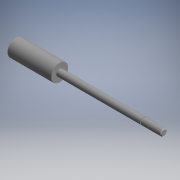
# Autodesk Inventor part: 0070.725-R0000_rod
Saved by Autodesk Inventor 2017.3 (Build 213256000, 256)
## iProperties
Part Number: 0070.725-R0000_rod
Material: Generic
Catalog Web Link: www.cadenas.de
Description: Standard Air Cylinder_rod-Original Line - Standard Air Cylinders
Vendor: BIMBA
Document SubType Name: Modeling
Designer: partserver
Manufacturer: BIMBA
Mass: 1.45088 g
Surface Area: 11.2381 cm^2
Volume: 1.45088 cm^3
Density: 1 g/cm^3
Appearance: PSOLRGB-181-181-181
Category: PARTsolutions
Company: BIMBA
Title: 0070.725-R0000_rod
Author: Cadenas PARTsolutions
Comments: Original Line - Standard Air Cylinders
PSOL_IDENT_0: {$CADENAS_DATA\23d-libs\bimba\bimba_brand\bimba_imperial\bimba_full_line\original_line_cylinders\sta
PSOL_IDENT_1: ndard_air_cylinders\rod.prj},337 {VTYP=3D},{NB=0070.725-R0000_rod},{LINA=0070.725-R0000_rod},{NN=Sta
PSOL_IDENT_2: ndard Air Cylinder_rod},{DATE=19.01.2022 10:19:37},{GEOMDATE=27.08.2019 11:00:52},{VERSION=},{LINEID=
PSOL_IDENT_3: 20},{WBVAR=STROKE,ACTING,MNT,DER,NR,BM,CO,M,EE,EEL,K,Q,Y,F,G,T,B,H,SER,SR,NT,W,E,HL,ST,STP,PRC,PB,CO
PSOL_IDENT_4: LOR1,FCD,RCD,BCD,ZHJ},{WBNUMERIC=STROKE,EEL,COLOR1,FCD,RCD,BCD,ZHJ}  {NB=0070.725-R0000_rod},{LINA=0
PSOL_IDENT_5: 070.725-R0000_rod},{KT=DUMMY},{PN=0070.725-R000},{DASH=-},{BORE=0.31250000},{BOREPN=007},{STROKE=0.7
PSOL_IDENT_6: 25},{STROKEALG=[0.001:50/0.001]},{STROKE1=0.725},{ACTING=R},{ACTINGALG= '' , 'Single Acting' , 'R' ,
PSOL_IDENT_7: 'Reverse Single Acting' , 'D' , 'Double Acting' },{ACTINGPN=R},{MNT=},{MNTALG= '' , 'Front Nose Mou
PSOL_IDENT_8: nting' , 'P' , 'Rear Pivot Mounting' },{TYPE=},{MNTPN=},{DER=},{DERALG= '' , 'N/A' },{NR=},{NRALG= ''
PSOL_IDENT_9: , 'N/A' },{NRPN=},{BM=},{BMALG= '' , 'N/A' },{BMPN=},{CO=},{COALG= '' , 'N/A' },{M=},{MALG= '', 'Wi
PSOL_IDENT_10: thout Magnet', 'M', 'With Magnet' },{EE=},{EEL=0},{EEMAX=49},{EEALG= '', 'Without Extra Extension', '
PSOL_IDENT_11: EE', 'With Extra Extension' },{EELALG=0},{EEPN=},{EEPN1=0.000},{K=},{KALG= '' , 'N/A' },{KPN=},{Q=},
PSOL_IDENT_12: {QALG= '' , 'Without Side Ported Rear Head' , 'Q' , 'With Side Ported Rear Head' },{QPN=},{Y=},{YALG=
PSOL_IDENT_13: '' , 'N/A' },{YPN=},{F=},{FALG= '', 'Standard', 'F', 'Molycoated Body' },{FPN=},{G=},{GPN=},{T=},{T
PSOL_IDENT_14: ALG= '' , 'Standard' , 'N' , 'Low Temperature' , 'V' , 'High Temperature' },{NPN=},{VPN=},{B=},{BALG=
PSOL_IDENT_15: '' , 'With Bumper' },{BPN=},{H=},{HALG= '', 'N/A' },{HPN=},{SER=},{SERALG= '' , 'N/A' },{SR=},{SRAL
PSOL_IDENT_16: G= 'C' , 'Carbon Steel Rod' , 'SR' , '303 Stainless Steel Rod' , '' , '303 Stainless Steel Rod1' },{
PSOL_IDENT_17: SRPN=},{SRCON=0},{NT=},{NTPN=},{W=},{WALG= '' , 'Without Wiper' , 'W' , 'With Wiper' },{WPN=},{E=},{
PSOL_IDENT_18: EALG= '' , 'Without Special Lube and Seals' , 'E' , 'With Special Lube and Seals' },{EPN=},{HL=},{HL
PSOL_IDENT_19: ALG= '' , 'N/A' },{ST=},{STALG= '' , 'Without Switch Track' , 'T' , 'With Switch Track' },{STP=},{ST
PSOL_IDENT_20: PALG= '' , 'N/A' },{STPN=},{PRC=},{PRCALG= '' , 'Without Piston Rod Clevis' , 'D-166-1' , 'With Pist
PSOL_IDENT_21: on Rod Clevis' },{PRCPN=},{PB=},{PBALG= '' , 'Without Pivot Bracket' , 'D-167' , 'With Pivot Bracket'
PSOL_IDENT_22: },{PBPN=},{TLEN=1.8150},{TEXT=0.148333},{SPACE=0.084762},{FRAC=3.4400},{RGCON=},{RGDACCON=R},{RHCON=
PSOL_IDENT_23: },{RHCONON=1},{RHACCON=R},{FNUTCON=1},{RNUTCON=0},{FNUTPN=D-801},{RNUTPN=},{FNUTTRANS=0.0000},{RNUTT
PSOL_IDENT_24: RANS=0.0000},{VHOLECON=0},{A1=0.8450},{A1N=0.6250},{A1P=0.8450},{A1B=0.9060},{A4=0.1585},{A4N=0.2550
PSOL_IDENT_25: },{A4P=0.1585},{A5=0.0220},{A1H=0.328},{A1NH=0.3280},{A1PH=0.8750},{A1BH=0.0000},{A1SH=0.0000},{A2H=
PSOL_IDENT_26: 0.1585},{A2NH=0.1585},{LENGTH=1.4900},{LENGTH1=1.4900},{LENGTH2=1.6500},{MUL=1.8125},{MUL11=1.8125},
PSOL_IDENT_27: {MUL22=1.8125},{MUL33=1.0875},{MUL2=1.2500},{MUL211=1.2500},{MUL222=1.2500},{MUL233=0.7500},{SSS=1.4
PSOL_IDENT_28: 500},{RGLEN=0.7085},{RHLEN=0.1915},{SSS1=2.0000},{A13=0.7190},{THDLEN1=0.3800},{THD1=0.1250},{TAB=UN
PSOL_IDENT_29: C},{THDLEN=0.3800},{THD=0.1250},{OD=0.3215},{RODL=2.7670},{PL=0.8170},{RODDIA=0.1250},{HEX=0.0000},{
PSOL_IDENT_30: RODTRANS=0.7250},{G1=0.0000},{ON=0},{G5=0.0000},{DERLEN=1.9500},{THOLE=0.0000},{WF=0.0000},{BADD=0.0
PSOL_IDENT_31: 000},{MADD=0.0000},{NVADD=0.000},{JRADD=0.00000},{COLOR=0.71,0.71,0.71,0.00},{GROOVE=1},{HOL=0},{D7=
PSOL_IDENT_32: 0.1270},{H1=0.0000},{D1=0.6050},{D1RH=0.3590},{D1P=0.0000},{D1B=0.6050},{D1N=0.3590},{D1NRH=0.3590},
PSOL_IDENT_33: {D1BRH=0.0000},{D1PRH=0.4380},{BOZO=1},{HADD=0.000},{COLOR1=0},{DEFL=0.0000},{HEXL=0.0000},{SSADD=0.
PSOL_IDENT_34: 0000},{WFL=0.0000},{MOVE=0.0000},{PRCL2=0.18800},{PRCB=0.11000},{PRCTRANS=0.00000},{FCD=0},{RCD=0},{
PSOL_IDENT_35: BCD=0},{ZHJ=0.000}
NB: 0070.725-R0000_rod
NN: Standard Air Cylinder_rod
NT: Standard
NBSYN: $PN.$COLOR1._rod
LINA: 0070.725-R0000_rod
CATALOG: Bimba Products
PN: 0070.725-R000
BORE: 0.3125
BOREPN: 007
STROKE: 0.725
ACTING: Reverse Single Acting
MNT: Front Nose Mounting
DER: N/A
NR: N/A
BM: N/A
CO: N/A
M: Without Magnet
EE: Without Extra Extension
EEL: 0
K: N/A
Q: Without Side Ported Rear Head
Y: N/A
F: Standard
G: Without Magnalube Lubrication
T: Standard
B: With Bumper
H: N/A
SER: N/A
SR: 303 Stainless Steel Rod1
W: Without Wiper
E: Without Special Lube and Seals
HL: N/A
ST: Without Switch Track
STP: N/A
PRC: Without Piston Rod Clevis
PB: Without Pivot Bracket
A1N: 0.625
A1P: 0.845
A1B: 0.906
A4N: 0.255
A4P: 0.1585
A5: 0.022
A1NH: 0.328
A1PH: 0.875
A1BH: 0
A1SH: 0
A2NH: 0.1585
A13: 0.719
THDLEN1: 0.38
THD1: 0.125
TAB: UNC
OD: 0.3215
RODDIA: 0.125
HEX: 0
G1: 0
G5: 0
THOLE: 0
WF: 0
GROOVE: 1
D7: 0.127
D1P: 0
D1B: 0.605
D1N: 0.359
D1NRH: 0.359
D1BRH: 0
D1PRH: 0.438
COLOR1: 0
FCD: 0
RCD: 0
BCD: 0
ZHJ: 0
SUPPLIER: BIMBA
ARTICLENO: 0070.725-R0000_rod
BOMINFO: 0070.725-R0000_rod
CREATOR: CADENAS GmbH
Autodesk Inventor part; units mm, degrees
sketch "Sketch_1" plane through (0, 0, 0) normal (0, 0, 1) x (1, 0, 0)
  line L0 (60.6298, 0) -> (0, 0)
  line L1 (0, 0) -> (0, 1.5875)
  line L2 (0, 1.5875) -> (39.878, 1.5875)
  line L3 (39.878, 1.5875) -> (39.878, 4.0323)
  line L4 (39.878, 4.0323) -> (60.6298, 4.0323)
  line L5 (60.6298, 4.0323) -> (60.6298, 0)
  line L6 (60.6298, 0) -> (0, 0)
  constraints: 14 end point
revolve "Revolution1" add sketch "Sketch_1" angle 360 about axis through (60.6298, 0, 0) along (1, 0, 0)
sketch "Sketch_2" plane through (0, 0, 0) normal (0, 0, 1) x (1, 0, 0)
  line L0 (0, 0) -> (-9.652, 0)
  line L1 (-9.652, 0) -> (-9.652, 1.209)
  line L2 (-9.652, 1.209) -> (-9.2735, 1.5875)
  line L3 (-9.2735, 1.5875) -> (0, 1.5875)
  line L4 (0, 1.5875) -> (0, 0)
  line L5 (0, 0) -> (-9.652, 0)
  constraints: 12 end point
revolve "Revolution2" add sketch "Sketch_2" angle 360 about axis through (0, 0, 0) along (1, 0, 0)
sketch "Sketch_30" plane through (0, 0, 0) normal (0, 0, 1) x (1, 0, 0)
  line L0 (0, 0) -> (-0.254, 0)
  line L1 (-0.254, 1.3335) -> (0, 1.3335)
  line L2 (0, 1.3335) -> (0, 1.8415)
  line L3 (0, 1.8415) -> (-0.254, 1.8415)
  line L4 (-0.254, 1.8415) -> (-0.254, 1.3335)
  constraints: 10 end point
revolve "Revolution3" cut sketch "Sketch_30" angle 360 about axis through (0, 0, 0) along (1, 0, 0)
ref_plane "dia1_XY" through (0, 1.5875, 0) normal (1, 0, 0) x (0, 0, -1)
ref_plane "dia1_YZ" through (0, 1.5875, 0) normal (0, 0, -1) x (0, 1, 0)
ref_plane "dia1_ZX" through (0, 1.5875, 0) normal (0, 1, 0) x (1, 0, 0)
ref_plane "dia12_XY" through (0, 0, 7.6835) normal (1, 0, 0) x (0, 0, -1)
ref_plane "dia12_YZ" through (0, 0, 7.6835) normal (0, 0, -1) x (0, 1, 0)
ref_plane "dia12_ZX" through (0, 0, 7.6835) normal (0, 1, 0) x (1, 0, 0)
ref_plane "dia1r_XY" through (0, 0, 4.5593) normal (1, 0, 0) x (0, 0, -1)
ref_plane "dia1r_YZ" through (0, 0, 4.5593) normal (0, 0, -1) x (0, 1, 0)
ref_plane "dia1r_ZX" through (0, 0, 4.5593) normal (0, 1, 0) x (1, 0, 0)
ref_plane "dia2_XY" through (0, -1.5875, 0) normal (1, 0, 0) x (0, 0, -1)
ref_plane "dia2_YZ" through (0, -1.5875, 0) normal (0, 0, -1) x (0, 1, 0)
ref_plane "dia2_ZX" through (0, -1.5875, 0) normal (0, 1, 0) x (1, 0, 0)
ref_plane "dia22_XY" through (0, 0, -7.6835) normal (1, 0, 0) x (0, 0, -1)
ref_plane "dia22_YZ" through (0, 0, -7.6835) normal (0, 0, -1) x (0, 1, 0)
ref_plane "dia22_ZX" through (0, 0, -7.6835) normal (0, 1, 0) x (1, 0, 0)
ref_plane "dia2r_XY" through (0, 0, -4.5593) normal (1, 0, 0) x (0, 0, -1)
ref_plane "dia2r_YZ" through (0, 0, -4.5593) normal (0, 0, -1) x (0, 1, 0)
ref_plane "dia2r_ZX" through (0, 0, -4.5593) normal (0, 1, 0) x (1, 0, 0)
ref_plane "rl1_XY" through (-9.652, 0, 0) normal (1, 0, 0) x (0, 0, -1)
ref_plane "rl1_YZ" through (-9.652, 0, 0) normal (0, 0, -1) x (0, 1, 0)
ref_plane "rl1_ZX" through (-9.652, 0, 0) normal (0, 1, 0) x (1, 0, 0)
ref_plane "rl2_XY" through (0, 0, 0) normal (1, 0, 0) x (0, 0, -1)
ref_plane "rl2_YZ" through (0, 0, 0) normal (0, 0, -1) x (0, 1, 0)
ref_plane "rl2_ZX" through (0, 0, 0) normal (0, 1, 0) x (1, 0, 0)
ref_plane "rod_cp_XY" through (0, 0, 0) normal (1, 0, 0) x (0, 0, -1)
ref_plane "rod_cp_YZ" through (0, 0, 0) normal (0, 0, -1) x (0, 1, 0)
ref_plane "rod_cp_ZX" through (0, 0, 0) normal (0, 1, 0) x (1, 0, 0)
ref_plane "stroke1_XY" through (0, 0, 0) normal (1, 0, 0) x (0, 0, -1)
ref_plane "stroke1_YZ" through (0, 0, 0) normal (0, 0, -1) x (0, 1, 0)
ref_plane "stroke1_ZX" through (0, 0, 0) normal (0, 1, 0) x (1, 0, 0)
ref_plane "thd1_XY" through (-9.652, 1.5875, 0) normal (1, 0, 0) x (0, 0, -1)
ref_plane "thd1_YZ" through (-9.652, 1.5875, 0) normal (0, 0, -1) x (0, 1, 0)
ref_plane "thd1_ZX" through (-9.652, 1.5875, 0) normal (0, 1, 0) x (1, 0, 0)
ref_plane "thd2_XY" through (-9.652, -1.5875, 0) normal (1, 0, 0) x (0, 0, -1)
ref_plane "thd2_YZ" through (-9.652, -1.5875, 0) normal (0, 0, -1) x (0, 1, 0)
ref_plane "thd2_ZX" through (-9.652, -1.5875, 0) normal (0, 1, 0) x (1, 0, 0)
ref_plane "to_rod_clevis_XY" through (-9.652, 0, 0) normal (1, 0, 0) x (0, 0, -1)
ref_plane "to_rod_clevis_YZ" through (-9.652, 0, 0) normal (0, 0, -1) x (0, 1, 0)
ref_plane "to_rod_clevis_ZX" through (-9.652, 0, 0) normal (0, 1, 0) x (1, 0, 0)
body "Solid1"
